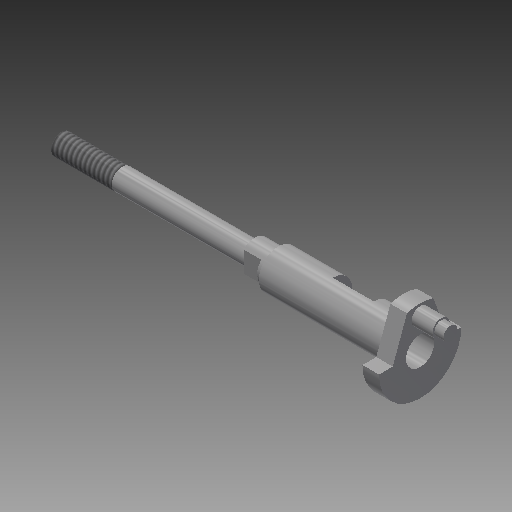
# Autodesk Inventor part: Crankshaft
Saved by Autodesk Inventor 2017 (Build 210135000, 135)
## iProperties
Created: 2012-08-06
Part Number: Crankshaft
Material: Steel
Document SubType Name: Modeling
Designer: John
Mass: 19.2188 g
Surface Area: 23.3403 cm^2
Volume: 2.44826 cm^3
Density: 7.85 g/cm^3
Appearance: Steel
Author: John
Autodesk Inventor part; units mm, degrees
ref_plane "YZ Plane" through (0, 0, 0) normal (1, 0, 0) x (0, 1, 0)
ref_plane "XZ Plane" through (0, 0, 0) normal (0, 1, 0) x (-1, 0, 0)
ref_plane "XY Plane" through (0, 0, 0) normal (0, 0, 1) x (1, 0, 0)
sketch "Sketch1" plane through (0, 0, 0) normal (1, 0, 0) x (0, 1, 0)
  circle A0 centre (0, 0) radius 9.4742
  dimension "d0" = 9.4742
  constraints: 1 centre point, 1 coincident
  measures "d0" radius of A0
extrude "Extrusion1" add sketch "Sketch1" against normal blind 3.81
sketch "Sketch2" plane through (0, 0, 0) normal (1, 0, 0) x (0, 0, -1)
  circle A0 centre (0, 0) radius 9.4742 projected
  circle A1 centre (0, 0) radius 4.5085
  dimension "d4" = 9.017
  constraints: 1 centre point, 1 coincident
  measures "d4" diameter of A1
extrude "Extrusion2" add sketch "Sketch2" against normal blind 32.639 contours A1
sketch "Sketch3" plane through (0, 0, 0) normal (1, 0, 0) x (0, 0, -1)
  circle A0 centre (0, 0) radius 9.4742 projected
  circle A1 centre (0, 0) radius 3.4925
  dimension "d9" = 6.985
  constraints: 1 centre point, 1 coincident
  measures "d9" diameter of A1
extrude "Extrusion3" add sketch "Sketch3" against normal blind 38.1 contours A1
sketch "Sketch4" plane through (0, 0, 0) normal (1, 0, 0) x (0, 0, -1)
  circle A0 centre (0, 0) radius 9.4742 projected
  circle A1 centre (0, 0) radius 2.413
  dimension "d13" = 4.826
  constraints: 1 centre point, 1 coincident
  measures "d13" diameter of A1
extrude "Extrusion4" add sketch "Sketch4" against normal blind 82.55 contours A1
sketch "Sketch5" plane through (0, 0, 0) normal (0, 0, 1) x (1, 0, 0)
  line L0 (-3.81, 9.4742) -> (0, 9.4742) projected
  line L1 (0, 9.4742) -> (0, -9.4742) projected
  line L2 (0, -9.4742) -> (-3.81, -9.4742) projected
  line L3 (-3.81, -9.4742) -> (-3.81, -4.5085) projected
  line L4 (-3.81, -4.5085) -> (-32.639, -4.5085) projected
  line L5 (-32.639, -4.5085) -> (-32.639, -3.4925) projected
  line L6 (-32.639, -3.4925) -> (-38.1, -3.4925) projected
  line L7 (-38.1, -3.4925) -> (-38.1, -2.413) projected
  line L8 (-38.1, -2.413) -> (-82.55, -2.413) projected
  line L9 (-82.55, -2.413) -> (-82.55, 2.413) projected
  line L10 (-82.55, 2.413) -> (-38.1, 2.413) projected
  line L11 (-38.1, 2.413) -> (-38.1, 3.4925) projected
  line L12 (-38.1, 3.4925) -> (-32.639, 3.4925) projected
  line L13 (-32.639, 3.4925) -> (-32.639, 4.5085) projected
  line L14 (-32.639, 4.5085) -> (-3.81, 4.5085) projected
  line L15 (-3.81, 4.5085) -> (-3.81, 9.4742) projected
  line L16 (-38.1, 3.4925) -> (-34.036, 3.4925)
  line L17 (-34.036, 3.4925) -> (-34.036, 2.54)
  line L18 (-34.036, 2.54) -> (-38.1, 2.54)
  line L19 (-38.1, 2.54) -> (-38.1, 3.4925)
  line L20 (-38.1, -3.4925) -> (-34.036, -3.4925)
  line L21 (-34.036, -3.4925) -> (-34.036, -2.54)
  line L22 (-34.036, -2.54) -> (-38.1, -2.54)
  line L23 (-38.1, -2.54) -> (-38.1, -3.4925)
  point P0 (0, 0)
  dimension "d17" = 34.036
  dimension "d18" = 5.08
  constraints: 16 end point, 4 parallel, 2 collinear, 2 horizontal, 2 perpendicular
  measures "d17" distance between parallel lines of L1 L17
  measures "d18" distance between parallel lines of L22 L18
extrude "Extrusion5" cut sketch "Sketch5" along normal through all both and the other way through all contours L17 L18 L11 L12 | L6 L7 L22 L21
thread "Thread1" size "10-24 UNC" class "2A" standard "ANSI Unified Screw Threads" length 13.97
sketch "Sketch6" plane through (0, 0, 0) normal (1, 0, 0) x (0, 0, -1)
  circle A0 centre (0, 0) radius 9.4742 projected
hole "Hole1" at (0, 0, 0) direction (-1, 0, 0) diameter 6.5278 depth 22.352
sketch "Sketch7" plane through (0, 0, 0) normal (0, 0, 1) x (1, 0, 0)
  line L0 (-3.81, 9.4742) -> (0, 9.4742) projected
  line L1 (0, 9.4742) -> (0, 3.2639) projected
  line L2 (0, 3.2639) -> (-22.352, 3.2639) projected
  line L3 (-22.352, 3.2639) -> (-22.352, -3.2639) projected
  line L4 (-22.352, -3.2639) -> (0, -3.2639) projected
  line L5 (0, -3.2639) -> (0, -9.4742) projected
  line L6 (0, -9.4742) -> (-3.81, -9.4742) projected
  line L7 (-3.81, -9.4742) -> (-3.81, -4.5085) projected
  line L8 (-3.81, -4.5085) -> (-32.639, -4.5085) projected
  line L9 (-32.639, -4.5085) -> (-32.639, -3.4925) projected
  line L10 (-32.639, -3.4925) -> (-34.036, -3.4925) projected
  line L11 (-34.036, -3.4925) -> (-34.036, -2.54) projected
  line L12 (-34.036, -2.54) -> (-38.1, -2.54) projected
  line L13 (-38.1, -2.54) -> (-38.1, -2.413) projected
  line L14 (-38.1, -2.413) -> (-82.55, -2.413) projected
  line L15 (-82.55, -2.413) -> (-82.55, 2.413) projected
  line L16 (-82.55, 2.413) -> (-38.1, 2.413) projected
  line L17 (-38.1, 2.413) -> (-38.1, 2.54) projected
  line L18 (-38.1, 2.54) -> (-34.036, 2.54) projected
  line L19 (-34.036, 2.54) -> (-34.036, 3.4925) projected
  line L20 (-34.036, 3.4925) -> (-32.639, 3.4925) projected
  line L21 (-32.639, 3.4925) -> (-32.639, 4.5085) projected
  line L22 (-32.639, 4.5085) -> (-3.81, 4.5085) projected
  line L23 (-3.81, 4.5085) -> (-3.81, 9.4742) projected
  line L24 (-65.532, 0) -> (10.922, 0) projected
  line L25 (-10.668, 0) -> (-20.1168, 0)
  line L26 (-20.1168, 0) -> (-20.1168, 4.5085)
  line L27 (-20.1168, 4.5085) -> (-10.668, 4.5085)
  line L28 (-10.668, 4.5085) -> (-10.668, 0)
  point P0 (0, 0)
  dimension "d30" = 10.668
  dimension "d31" = 20.1168
  constraints: 8 end point, 2 parallel, 2 point on line, 1 horizontal, 1 perpendicular
  measures "d30" distance between parallel lines of L1 L28
  measures "d31" distance between parallel lines of L1 L26
extrude "Extrusion6" cut sketch "Sketch7" along normal through all contours L28 L2 L26 L22 | L28 L24 L26 L2
sketch "Sketch8" plane through (0, 0, 0) normal (1, 0, 0) x (0, 0, -1)
  circle A0 centre (0, 0) radius 3.2639 projected
  circle A1 centre (0, 0) radius 9.4742 projected
  line L0 (0, -9.4742) -> (0, -6.2992)
  line L1 (0, -6.2992) -> (-8.9758, -3.0323)
  line L2 (0, 0) -> (-9.4742, 0)
  line L3 (0, 9.4742) -> (0, 6.2992)
  line L4 (0, 6.2992) -> (-8.9758, 3.0323)
  dimension "d34" = 3.175
  dimension "d36" = 110
  constraints: 10 end point, 5 point on circle, 2 perpendicular, 1 collinear, 1 vertical, 1 vertical alignment, 1 other
  measures "d34" distance of L0.start L0.end
  measures "d36" angle of L1 L0
extrude "Extrusion7" cut sketch "Sketch8" against normal through all contours A1 L3 L4 | L1 L0 A1
sketch "Sketch9" plane through (0, 0, 0) normal (1, 0, 0) x (0, 0, -1)
  arc A0 (0, -9.4742) -> (0, 9.4742) centre (0, 0) ccw projected
  circle A1 centre (-6.9342, 0) radius 1.9939
  dimension "d43" = 6.9342
  dimension "d47" = 3.9878
  constraints: 1 centre point
  measures "d43" distance of A0.centre A1.centre
  measures "d47" diameter of A1
extrude "Extrusion8" add sketch "Sketch9" along normal blind 4.826
sketch "Sketch10" plane through (4.826, 0, 6.9342) normal (1, 0, 0) x (0, 0, -1)
  circle A0 centre (0, 0) radius 1.9939 projected
  circle A1 centre (0, 0) radius 1.5875
  point P0 (6.9342, 0)
  dimension "d49" = 3.175
  constraints: 1 centre point, 1 coincident
  measures "d49" diameter of A1
extrude "Extrusion9" add sketch "Sketch10" along normal blind 2.159 contours A1
body "Solid1"
